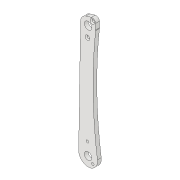
# Autodesk Inventor part: COXA_ROLL_LONG-LINK
Saved by Autodesk Inventor 2019.4 (Build 234330000, 330)
## iProperties
Created: 2019-10-21
Part Number: COXA_ROLL_LONG-LINK
Material: 一般
Document SubType Name: Modeling
Designer: y6tada
Density: 1 g/cm^3
Appearance: 白
Author: y6tada
Autodesk Inventor part; units mm, degrees
ref_plane "YZ Plane" through (0, 0, 0) normal (1, 0, 0) x (0, 1, 0)
ref_plane "XZ Plane" through (0, 0, 0) normal (0, 1, 0) x (-1, 0, 0)
ref_plane "XY Plane" through (0, 0, 0) normal (0, 0, 1) x (1, 0, 0)
sketch "スケッチ1" plane through (0, 0, 0) normal (0, 0, 1) x (1, 0, 0)
  line L0 (0, 0) -> (0, -60) construction
  arc A0 (0, -4) -> (3.9768, -0.4299) centre (0, 0) ccw construction
  arc A1 (0, -55) -> (-4.9993, -59.9167) centre (0, -60) ccw construction
  arc A2 (3.9768, -0.4299) -> (4.9505, -59.2985) centre (240.1879, -25.9652) ccw
  arc A3 (-3.9994, 0.0667) -> (0, -4) centre (0, 0) ccw construction
  arc A4 (3.9768, -0.4299) -> (4, 0) centre (0, 0) ccw
  arc A5 (4.9505, -59.2985) -> (0, -55) centre (0, -60) ccw construction
  arc A6 (-4.9993, -59.9167) -> (4.9505, -59.2985) centre (0, -60) ccw
  line L1 (-3.9994, 0.0667) -> (-4.9993, -59.9167)
  line L2 (2.6336, -22.0054) -> (2.3154, -41.0967) construction
  circle A7 centre (0, 0) radius 2 construction
  line L3 (-1.12, 3.84) -> (1.76, 4.68)
  line L4 (4, 3) -> (4, 0)
  arc A8 (4, 3) -> (1.76, 4.68) centre (2.25, 3) ccw
  circle A9 centre (2.25, 3) radius 1 construction
  arc A10 (-1.12, 3.84) -> (-3.9994, 0.0667) centre (0, 0) ccw
  arc A11 (4, 0) -> (-1.12, 3.84) centre (0, 0) ccw construction
  circle A12 centre (2.25, 3) radius 1.75 construction
  line L5 (-0.3242, -5.7627) -> (0, 0) construction
  circle A13 centre (-0.3242, -5.7627) radius 3.7718 construction
  circle A14 centre (0, -60) radius 2 construction
  circle A15 centre (0, -60) radius 3.5 construction
  line L6 (0, -60) -> (2.4749, -62.4749) construction
  circle A16 centre (-0.3611, -53.4798) radius 4.5302 construction
  dimension "d26" = 7
  dimension "d0" = 60
  dimension "d1" = 4
  dimension "d2" = 5
  dimension "d14" = 7
  dimension "d15" = 4
  dimension "d16" = 1.75
  dimension "d17" = 2
  dimension "d25" = 4
  dimension "d27" = 45
  constraints: 22 point on circle, 21 tangent, 16 centre point, 14 end point, 12 coincident, 2 point on line, 2 vertical, 1 concentric, 1 parallel, 3 other
  measures "d0" distance of L0.start L0.end
  measures "d1" radius of A4
  measures "d2" radius of A6
  measures "d14" distance between parallel lines of L2 L1
  measures "d15" diameter of A7
  measures "d16" radius of A8
  measures "d17" diameter of A9
  measures "d25" diameter of A14
  measures "d27" angle of L0 L6
extrude "押し出し1" add sketch "スケッチ1" along normal blind 2
hole "穴1" at (0, 0, 0) at (0, -60, 0) direction (0, 0, 1) diameter 4 end through all
hole "穴2" at (-0.3611, -53.4798, 0) at (2.4749, -62.4749, 0) direction (0, 0, 1) diameter 1.4 end through all countersink diameter 2.5 countersink angle 90
sketch "スケッチ2" plane through (0, 0, 2) normal (0, 0, 1) x (1, 0, 0)
  point P0 (0, 0)
  point P1 (2.25, 3)
  point P2 (-0.3242, -5.7627)
hole "穴4" at (2.25, 3, 2) at (-0.3242, -5.7627, 2) direction (0, 0, -1) diameter 1.4 end through all countersink diameter 2.5 countersink angle 90
